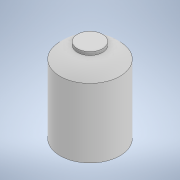
# Autodesk Inventor part: DuraCast_V325Gallon
Saved by Autodesk Inventor 2022 (Build 260153000, 153)
## iProperties
Created: 2021-06-29
Part Number: DuraCast_V325Gallon
Material: Generic
Document SubType Name: Modeling
Designer: jamieson-bl
Density: 1 g/cm^3
Appearance: Default
Author: jamieson-bl
Autodesk Inventor part; units mm, degrees
ref_plane "YZ Plane" through (0, 0, 0) normal (1, 0, 0) x (0, 1, 0)
ref_plane "XZ Plane" through (0, 0, 0) normal (0, 1, 0) x (-1, 0, 0)
ref_plane "XY Plane" through (0, 0, 0) normal (0, 0, 1) x (1, 0, 0)
sketch "Sketch1" plane through (0, 0, 0) normal (0, 0, 1) x (1, 0, 0)
  line L0 (0, -628.396) -> (-546.1, -628.396)
  line L1 (-546.1, -628.396) -> (-546.1, 628.396)
  line L2 (-546.1, 628.396) -> (0, 628.396)
  line L3 (546.1, -628.396) -> (-546.1, 628.396) construction
  line L4 (-546.1, -628.396) -> (546.1, 628.396) construction
  line L5 (0, 905.764) -> (-228.6, 905.764)
  line L6 (-228.6, 905.764) -> (-228.6, 846.328)
  line L7 (-228.6, 846.328) -> (0, 846.328)
  line L8 (228.6, 846.328) -> (228.6, 847.5028)
  line L9 (0, 876.046) -> (-228.6, 846.328) construction
  line L10 (-228.6, 905.764) -> (0, 876.046) construction
  arc A0 (-228.6, 846.328) -> (-546.1, 628.396) centre (1.7381, 170.5087) ccw
  line L11 (0, 905.764) -> (0, -628.396)
  point P0 (0, 0)
  dimension "d0" = 1092.2
  dimension "d1" = 1256.792
  dimension "d2" = 457.2
  dimension "d3" = 59.436
  dimension "d4" = 713.994
  constraints: 24 end point, 3 parallel, 3 point on circle, 3 point on line, 2 horizontal, 2 midpoint, 2 perpendicular, 1 centre point
  measures "d0" distance of L1.end L4.end
  measures "d1" distance of L0.end L1.end
  measures "d2" distance of L8.start L6.end
  measures "d3" distance of L6.end L5.end
  measures "d4" radius of A0
revolve "Revolution1" add sketch "Sketch1" angle 360 about axis through (0, 905.764, 0) along (0, 1, 0)
body "Solid1"
